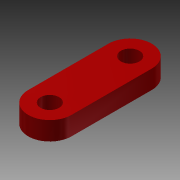
# Autodesk Inventor part: plastic_part_13
Saved by Autodesk Inventor 2013 (Build 170138000, 138)
## iProperties
Shininess: 20.0
Created: 2014-03-04
Part Number: plastic_part_13
Document SubType Name: Modeling
Designer: Noa Izumi
Material: Default
Density: 1 g/cm^3
Density: 0.0
Volumn: 0.0
Area: 0.0
PropertySet Name: Model Information
Control State: 0
Master: False
Checked Out: False
Author: Noa Izumi
Autodesk Inventor part; units mm, degrees
ref_plane "YZ Plane" through (0, 0, 0) normal (1, 0, 0) x (0, 1, 0)
ref_plane "XZ Plane" through (0, 0, 0) normal (0, 1, 0) x (-1, 0, 0)
ref_plane "XY Plane" through (0, 0, 0) normal (0, 0, 1) x (1, 0, 0)
sketch "Sketch1" plane through (0, 0, 0) normal (0, 0, 1) x (1, 0, 0)
  line L0 (0, 0) -> (7, 0)
  line L1 (7, 0) -> (7, 20)
  line L2 (7, 20) -> (0, 20)
  line L3 (0, 20) -> (0, 0)
  dimension "d0" = 7
  dimension "d1" = 20
  constraints: 8 end point, 2 parallel, 1 horizontal, 1 perpendicular
  measures "d0" distance of L0.start L0.end
  measures "d1" distance of L2.end L0.start
extrude "Extrusion1" add sketch "Sketch1" along normal blind 3
fillet "Fillet1" radius 3.5 4 edges at (0, 0, 1.5) (7, 0, 1.5) (0, 20, 1.5) (7, 20, 1.5)
sketch "Sketch2" plane through (0, 0, 3) normal (0, 0, 1) x (1, 0, 0)
  arc A0 (7, 16.5) -> (0, 16.5) centre (3.5, 16.5) ccw projected
  arc A1 (0, 3.5) -> (7, 3.5) centre (3.5, 3.5) ccw projected
  constraints: 2 coincident
hole "Hole1" at (3.5, 3.5, 3) at (3.5, 16.5, 3) direction (0, 0, -1) diameter 3 end through all
